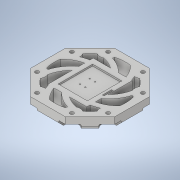
# Autodesk Inventor part: Bottom
Saved by Autodesk Inventor 2020 (Build 240168000, 168)
## iProperties
Created: 2018-10-03
Part Number: Bottom
Material: Generic
Document SubType Name: Modeling
Designer: isaac
Density: 1 g/cm^3
Appearance: Default
Author: isaac
Autodesk Inventor part; units mm, degrees
ref_plane "YZ Plane" through (0, 0, 0) normal (1, 0, 0) x (0, 1, 0)
ref_plane "XZ Plane" through (0, 0, 0) normal (0, 1, 0) x (-1, 0, 0)
ref_plane "XY Plane" through (0, 0, 0) normal (0, 0, 1) x (1, 0, 0)
sketch "Sketch1" plane through (0, 0, 0) normal (0, 1, 0) x (-1, 0, 0)
  circle A0 centre (0, 0) radius 88.9
  line L0 (82.1329, -34.0206) -> (34.0206, -82.1329)
  line L1 (34.0206, -82.1329) -> (-34.0206, -82.1329)
  line L2 (-34.0206, -82.1329) -> (-82.1329, -34.0206)
  line L3 (-82.1329, -34.0206) -> (-82.1329, 34.0206)
  line L4 (-82.1329, 34.0206) -> (-34.0206, 82.1329)
  line L5 (-34.0206, 82.1329) -> (34.0206, 82.1329)
  line L6 (34.0206, 82.1329) -> (82.1329, 34.0206)
  line L7 (82.1329, 34.0206) -> (82.1329, -34.0206)
  line L8 (0, 0) -> (105.0624, 0)
  line L9 (0, 0) -> (82.1329, 0)
  dimension "d0" = 177.8
  dimension "d1" = 68.0411
  constraints: 20 end point, 2 coincident, 1 collinear, 1 horizontal, 1 midpoint, 20 other
  measures "d1" distance of L0.end L1.end
extrude "Extrusion1" add sketch "Sketch1" along normal blind 25.4 contours L7 L0 L1 L2 L3 L4 L5 L6
sketch "Sketch31" plane through (0, 25.4, 0) normal (0, 1, 0) x (1, 0, 0)
  circle A0 centre (34.0206, 69.4329) radius 3.6195
  line L0 (34.0206, 82.1329) -> (-34.0206, 82.1329) projected
  line L1 (0, 0) -> (89.8026, 89.8026)
  line L2 (0, 0) -> (127, 0) construction
  circle A1 centre (69.4329, 34.0206) radius 3.6195
  circle A2 centre (-69.4329, 34.0206) radius 3.6195
  circle A3 centre (-34.0206, 69.4329) radius 3.6195
  circle A4 centre (-34.0206, -69.4329) radius 3.6195
  circle A5 centre (-69.4329, -34.0206) radius 3.6195
  circle A6 centre (69.4329, -34.0206) radius 3.6195
  circle A7 centre (34.0206, -69.4329) radius 3.6195
  dimension "d212" = 7.239
  dimension "d213" = 12.7
  dimension "d214" = 0
  dimension "d215" = 127
  dimension "d216" = 45
  dimension "d219" = 360
  constraints: 8 centre point, 4 end point, 1 equal length, 1 horizontal, 1 symmetric about line, 18 other
  measures "d212" diameter of A0
  measures "d213" distance from line of L0 A0.centre
  measures "d214" horizontal distance of L0.start A0.centre
  measures "d215" distance of L1.start L1.end
  measures "d216" angle of L2 L1
chamfer "Chamfer17" distance 8.89 angle 45 9 edges at (82.1329, 0, 0) (58.0767, 0, 58.0767) (0, 0, 82.1329) (-58.0767, 0, 58.0767) (-82.1329, 0, 17.0103) (-82.1329, 0, -17.0103) (-58.0767, 0, -58.0767) (0, 0, -82.1329) (58.0767, 0, -58.0767)
extrude "Extrusion26" cut sketch "Sketch31" against normal blind 25.4
sketch "Sketch32" plane through (0, 0, 0) normal (0, -1, 0) x (1, 0, 0)
  circle A0 centre (69.4329, 34.0206) radius 3.6195 projected
  circle A1 centre (69.4329, 34.0206) radius 12.7
  circle A2 centre (34.0206, 69.4329) radius 3.6195 projected
  circle A3 centre (34.0206, 69.4329) radius 12.7
  circle A4 centre (-34.0206, 69.4329) radius 12.7
  circle A5 centre (-69.4329, 34.0206) radius 12.7
  circle A6 centre (-69.4329, -34.0206) radius 12.7
  circle A7 centre (-34.0206, -69.4329) radius 12.7
  circle A8 centre (34.0206, -69.4329) radius 12.7
  circle A9 centre (69.4329, -34.0206) radius 12.7
  line L0 (69.4329, 21.3206) -> (90.8174, 21.3206)
  line L1 (36.643, 66.9381) -> (66.9381, 36.643) projected
  line L2 (60.5167, 43.0644) -> (77.7137, 60.0187)
  line L3 (77.7137, 60.0187) -> (96.7746, 43.8668)
  line L4 (96.7746, 43.8668) -> (90.8174, 21.3206)
  line L5 (43.0644, 60.5167) -> (60.2704, 77.969)
  line L6 (60.2704, 77.969) -> (26.119, 108.2881)
  line L7 (21.3206, 69.4329) -> (21.3206, 92.0788)
  line L8 (21.3206, 92.0788) -> (26.119, 108.2881)
  circle A10 centre (-34.0206, 69.4329) radius 12.7
  circle A11 centre (-69.4329, 34.0206) radius 12.7
  line L9 (-69.4329, 21.3206) -> (-92.0788, 21.3206)
  line L10 (-60.5167, 43.0644) -> (-77.969, 60.2704)
  line L11 (-92.0788, 21.3206) -> (-108.2881, 26.119)
  line L12 (-43.0644, 60.5167) -> (-60.0187, 77.7137)
  line L13 (-77.969, 60.2704) -> (-108.2881, 26.119)
  line L14 (-21.3206, 69.4329) -> (-21.3206, 90.8174)
  line L15 (-60.0187, 77.7137) -> (-43.8668, 96.7746)
  line L16 (-43.8668, 96.7746) -> (-21.3206, 90.8174)
  circle A12 centre (-69.4329, -34.0206) radius 12.7
  circle A13 centre (-34.0206, -69.4329) radius 12.7
  line L17 (-21.3206, -69.4329) -> (-21.3206, -92.0788)
  line L18 (-43.0644, -60.5167) -> (-60.2704, -77.969)
  line L19 (-21.3206, -92.0788) -> (-26.119, -108.2881)
  line L20 (-60.5167, -43.0644) -> (-77.7137, -60.0187)
  line L21 (-60.2704, -77.969) -> (-26.119, -108.2881)
  line L22 (-69.4329, -21.3206) -> (-90.8174, -21.3206)
  line L23 (-77.7137, -60.0187) -> (-96.7746, -43.8668)
  line L24 (-96.7746, -43.8668) -> (-90.8174, -21.3206)
  circle A14 centre (34.0206, -69.4329) radius 12.7
  circle A15 centre (69.4329, -34.0206) radius 12.7
  line L25 (69.4329, -21.3206) -> (92.0788, -21.3206)
  line L26 (60.5167, -43.0644) -> (77.969, -60.2704)
  line L27 (92.0788, -21.3206) -> (108.2881, -26.119)
  line L28 (43.0644, -60.5167) -> (60.0187, -77.7137)
  line L29 (77.969, -60.2704) -> (108.2881, -26.119)
  line L30 (21.3206, -69.4329) -> (21.3206, -90.8174)
  line L31 (60.0187, -77.7137) -> (43.8668, -96.7746)
  line L32 (43.8668, -96.7746) -> (21.3206, -90.8174)
  point P0 (0, 0)
  dimension "d226" = 25.4
  dimension "d227" = 25.4
  dimension "d230" = 360
  dimension "d291" = 360
  constraints: 64 end point, 16 point on circle, 14 centre point, 2 coincident, 2 point on line, 2 tangent, 1 horizontal, 1 vertical, 108 other
  measures "d226" diameter of A1
  measures "d227" diameter of A3
extrude "Extrusion27" cut sketch "Sketch32" against normal blind 12.7 contours A0 | A1 | A1 L2 L3 L4 L0 | A2 | A3 | A3 L7 L8 L6 L5 | A4 | A4 L12 L15 L16 L14 | A5 | A5 L9 L11 L13 L10 | A6 | A6 L20 L23 L24 L22 | A7 | L17 L19 L21 L18 A7 | A8 | A8 L28 L31 L32 L30 | A9 | A9 L25 L27 L29 L26
sketch "Sketch33" plane through (0, 25.4, 0) normal (0, 1, 0) x (1, 0, 0)
  line L0 (-28.575, 33.655) -> (28.575, 33.655)
  line L1 (28.575, 33.655) -> (28.575, -33.655)
  line L2 (28.575, -33.655) -> (-28.575, -33.655)
  line L3 (-28.575, -33.655) -> (-28.575, 33.655)
  line L4 (-28.575, 33.655) -> (28.575, -33.655) construction
  line L5 (28.575, 33.655) -> (-28.575, -33.655) construction
  point P0 (0, 0)
  dimension "d234" = 57.15
  dimension "d235" = 67.31
  constraints: 12 end point, 2 midpoint, 2 parallel, 1 horizontal, 1 perpendicular
  measures "d234" distance of L1.end L2.end
  measures "d235" distance of L0.end L1.end
extrude "Extrusion28" cut sketch "Sketch33" against normal blind 3.175
sketch "Sketch35" plane through (0, 25.4, 0) normal (0, 1, 0) x (1, 0, 0)
  line L0 (-82.1329, 34.0206) -> (-82.1329, -34.0206) projected
  line L1 (-34.0206, 82.1329) -> (-82.1329, 34.0206) projected
  line L2 (34.0206, 82.1329) -> (-34.0206, 82.1329) projected
  line L3 (49.3059, 66.8475) -> (66.8475, 49.3059) projected
  line L4 (82.1329, -34.0206) -> (82.1329, 34.0206) projected
  line L5 (66.8475, -49.3059) -> (49.3059, -66.8475) projected
  line L6 (21.3206, -82.1329) -> (-21.3206, -82.1329) projected
  line L7 (-49.3059, -66.8475) -> (-66.8475, -49.3059) projected
  arc A0 (-38.1, 9.1271) -> (-58.2083, -22.7945) centre (4.8156, -40.2008) ccw
  line L8 (-38.1, -44.45) -> (38.1, -44.45)
  line L9 (-38.1, -44.45) -> (38.1, 44.45) construction
  line L10 (38.1, -44.45) -> (-38.1, 44.45) construction
  arc A1 (2.7863, 44.45) -> (-22.7945, 58.2083) centre (-40.2008, -4.8156) ccw
  arc A2 (41.3, -6.1494) -> (58.2083, 22.7945) centre (-4.8156, 40.2008) ccw
  arc A3 (-2.7863, -44.45) -> (11.3195, -53.8433) centre (40.2008, 4.8156) ccw
  arc A4 (11.0921, 44.45) -> (-19.42, 63.2007) centre (-40.2008, -4.8156) ccw
  arc A5 (38.1, -16.5117) -> (63.2007, 19.42) centre (-4.8156, 40.2008) ccw
  arc A6 (-11.0921, -44.45) -> (19.42, -63.2007) centre (40.2008, 4.8156) ccw
  arc A7 (-38.1, 16.5117) -> (-63.2007, -19.42) centre (4.8156, -40.2008) ccw
  arc A8 (-38.1, 38.0757) -> (-53.574, 33.3053) centre (-25.0211, -31.8314) ccw
  arc A9 (36.5833, 44.45) -> (33.3053, 53.574) centre (-31.8314, 25.0211) ccw
  arc A10 (38.1, -38.0757) -> (53.574, -33.3053) centre (25.0211, 31.8314) ccw
  arc A11 (-36.5833, -44.45) -> (-33.3053, -53.574) centre (31.8314, -25.0211) ccw
  circle A12 centre (-69.4329, 34.0206) radius 3.6195 projected
  circle A13 centre (-34.0206, 69.4329) radius 3.6195 projected
  circle A14 centre (34.0206, 69.4329) radius 3.6195 projected
  circle A15 centre (69.4329, -34.0206) radius 3.6195 projected
  circle A16 centre (34.0206, -69.4329) radius 3.6195 projected
  circle A17 centre (-34.0206, -69.4329) radius 3.6195 projected
  circle A18 centre (-69.4329, -34.0206) radius 3.6195 projected
  arc A19 (25.9496, 44.45) -> (10.8089, 68.5864) centre (-31.8314, 25.0211) ccw
  arc A20 (38.1, -3.0933) -> (54.8559, 27.7335) centre (-4.8156, 40.2008) ccw
  arc A21 (38.1, -27.7091) -> (68.5864, -10.8089) centre (25.0211, 31.8314) ccw
  arc A22 (4.2978, -44.45) -> (27.7335, -54.8559) centre (40.2008, 4.8156) ccw
  arc A23 (-25.9496, -44.45) -> (-10.8089, -68.5864) centre (31.8314, -25.0211) ccw
  arc A24 (-38.1, 3.0933) -> (-54.8559, -27.7335) centre (4.8156, -40.2008) ccw
  arc A25 (-38.1, 27.7091) -> (-68.5864, 10.8089) centre (-25.0211, -31.8314) ccw
  arc A26 (-40.3622, 31.7268) -> (-55.8284, 25.8392) centre (-25.0211, -31.8314) ccw
  arc A27 (-66.9456, 18.3416) -> (-66.9727, 18.3189) centre (-25.0211, -31.8314) ccw
  arc A28 (-53.574, 33.3053) -> (-55.5293, 41.6825) centre (-69.4329, 34.0206) ccw
  arc A29 (-41.6825, 55.5293) -> (-55.5293, 41.6825) centre (0, 0) ccw
  arc A30 (-19.42, 63.2007) -> (-18.3382, 66.9674) centre (-34.0206, 69.4329) ccw
  arc A31 (-24.4956, 82.1329) -> (-49.6272, 66.5263) centre (-34.0206, 69.4329) ccw
  arc A32 (-41.6825, 55.5293) -> (-27.7335, 54.8559) centre (-34.0206, 69.4329) ccw
  arc A33 (-66.9674, 18.3382) -> (-66.9674, -18.3382) centre (0, 0) ccw
  arc A34 (-55.5293, -41.6825) -> (-66.9674, -18.3382) centre (-69.4329, -34.0206) ccw
  arc A35 (-82.1329, -24.4956) -> (-66.5263, -49.6272) centre (-69.4329, -34.0206) ccw
  arc A36 (-66.5263, 49.6272) -> (-82.1329, 24.4956) centre (-69.4329, 34.0206) ccw
  arc A37 (-66.9674, 18.3382) -> (-55.8284, 25.8392) centre (-69.4329, 34.0206) ccw
  arc A38 (-55.5293, -41.6825) -> (-41.6825, -55.5293) centre (0, 0) ccw
  arc A39 (-30.5986, -44.45) -> (-25.8392, -55.8284) centre (31.8314, -25.0211) ccw
  arc A40 (-18.3416, -66.9456) -> (-18.3189, -66.9727) centre (31.8314, -25.0211) ccw
  arc A41 (-49.6272, -66.5263) -> (-24.4956, -82.1329) centre (-34.0206, -69.4329) ccw
  arc A42 (-18.3382, -66.9674) -> (-18.3416, -66.9456) centre (-34.0206, -69.4329) ccw
  arc A43 (-33.3053, -53.574) -> (-41.6825, -55.5293) centre (-34.0206, -69.4329) ccw
  arc A44 (-18.3382, -66.9674) -> (-18.3189, -66.9727) centre (0, 0) ccw
  arc A45 (-10.8089, -68.5864) -> (18.3382, -66.9674) centre (0, 0) ccw
  arc A46 (24.4956, -82.1329) -> (49.6272, -66.5263) centre (34.0206, -69.4329) ccw
  arc A47 (41.6825, -55.5293) -> (27.7335, -54.8559) centre (34.0206, -69.4329) ccw
  arc A48 (19.42, -63.2007) -> (18.3382, -66.9674) centre (34.0206, -69.4329) ccw
  arc A49 (41.6825, -55.5293) -> (55.5293, -41.6825) centre (0, 0) ccw
  arc A50 (66.5263, -49.6272) -> (82.1329, -24.4956) centre (69.4329, -34.0206) ccw
  arc A51 (38.1, -32.2306) -> (55.8284, -25.8392) centre (25.0211, 31.8314) ccw
  arc A52 (66.9456, -18.3416) -> (66.9727, -18.3189) centre (25.0211, 31.8314) ccw
  line L11 (38.1, -44.45) -> (38.1, -38.0757)
  arc A53 (66.9674, -18.3382) -> (55.8284, -25.8392) centre (69.4329, -34.0206) ccw
  arc A54 (53.574, -33.3053) -> (55.5293, -41.6825) centre (69.4329, -34.0206) ccw
  arc A55 (66.9674, -18.3382) -> (66.9727, -18.3189) centre (0, 0) ccw
  arc A56 (68.5864, -10.8089) -> (66.9674, 18.3382) centre (0, 0) ccw
  arc A57 (63.2007, 19.42) -> (66.9674, 18.3382) centre (69.4329, 34.0206) ccw
  arc A58 (82.1329, 24.4956) -> (66.5263, 49.6272) centre (69.4329, 34.0206) ccw
  arc A59 (55.5293, 41.6825) -> (54.8559, 27.7335) centre (69.4329, 34.0206) ccw
  line L12 (38.1, -32.2306) -> (38.1, -16.5117)
  line L13 (38.1, -3.0933) -> (38.1, 44.45)
  arc A60 (55.5293, 41.6825) -> (41.6825, 55.5293) centre (0, 0) ccw
  arc A61 (18.3382, 66.9674) -> (-18.3382, 66.9674) centre (0, 0) ccw
  arc A62 (30.5986, 44.45) -> (25.8392, 55.8284) centre (-31.8314, 25.0211) ccw
  arc A63 (18.3416, 66.9456) -> (18.3189, 66.9727) centre (-31.8314, 25.0211) ccw
  arc A64 (49.6272, 66.5263) -> (24.4956, 82.1329) centre (34.0206, 69.4329) ccw
  arc A65 (18.3382, 66.9674) -> (41.6825, 55.5293) centre (34.0206, 69.4329) ccw
  arc A66 (-4.2978, 44.45) -> (-27.7335, 54.8559) centre (-40.2008, -4.8156) ccw
  line L14 (38.1, 44.45) -> (2.7863, 44.45)
  line L15 (-4.2978, 44.45) -> (-38.1, 44.45)
  line L16 (-38.1, 3.0933) -> (-38.1, -44.45)
  line L17 (-38.1, 44.45) -> (-38.1, 38.0757)
  line L18 (-38.1, 27.7091) -> (-38.1, 16.5117)
  point P0 (46.7206, 69.4329)
  point P1 (69.4329, 46.7206)
  point P2 (69.4329, -46.7206)
  point P3 (46.7206, -69.4329)
  point P4 (34.0206, -82.1329)
  point P5 (-34.0206, -82.1329)
  point P6 (-46.7206, -69.4329)
  point P7 (-69.4329, -46.7206)
  dimension "d250" = 76.2
  dimension "d251" = 88.9
  dimension "d254" = 71.12
  dimension "d255" = 71.12
  dimension "d257" = 71.12
  dimension "d259" = 71.12
  dimension "d268" = 60.96
  dimension "d269" = 60.96
  dimension "d270" = 60.96
  dimension "d271" = 60.96
  dimension "d272" = 60.96
  dimension "d273" = 60.96
  dimension "d274" = 60.96
  dimension "d275" = 60.96
  constraints: 135 point on circle, 60 centre point, 27 point on line, 24 coincident, 22 end point, 11 parallel, 3 perpendicular, 1 horizontal, 1 midpoint
  measures "d250" distance of L10.end L9.end
  measures "d251" distance of L9.end L8.end
  measures "d254" radius of A4
  measures "d255" radius of A5
  measures "d257" radius of A6
  measures "d259" radius of A7
  measures "d268" radius of A19
  measures "d269" radius of A20
  measures "d270" radius of A21
  measures "d271" radius of A22
  measures "d272" radius of A23
  measures "d273" radius of A24
  measures "d274" radius of A25
  measures "d275" radius of A66
extrude "Extrusion30" cut sketch "Sketch35" against normal through all contours L8 A11 A43 A38 A34 A24 L16 | L8 A6 A48 A45 A23 | L8 L11 A10 A54 A49 A47 A22 | A4 A30 A61 A19 L14 | A9 A65 A60 A59 A20 L13 L14 | A5 A57 A56 A21 L12 | A7 A34 A33 A25 L18 | A8 A28 A29 A32 A66 L15 L17
fillet "Fillet5" radius 1.5875 8 edges at (-57.6824, 12.7, 29.2022) (-29.2022, 12.7, 57.6824) (29.2022, 12.7, 57.6824) (57.6824, 12.7, 29.2022) (-57.6824, 12.7, -29.2022) (-29.2022, 12.7, -57.6824) (29.2022, 12.7, -57.6824) (57.6824, 12.7, -29.2022)
fillet "Fillet6" radius 6.35 8 edges at (53.4874, 0, 0.5277) (35.1, 0, -49.0679) (-2.9644, 0, -55.7774) (-45.9732, 0, -36.1323) (-53.4874, 0, -0.5277) (-35.1, 0, 49.0679) (2.9644, 0, 55.7774) (45.9732, 0, 36.1323)
sketch "Sketch37" plane through (0, 0, 0) normal (0, -1, 0) x (1, 0, 0)
  circle A0 centre (-10.0076, 9.4933) radius 1.0351 construction
  circle A1 centre (-10.0076, -9.4933) radius 1.0351 construction
  circle A2 centre (0.4572, -9.4933) radius 1.0351 construction
  circle A3 centre (0.4572, 9.4933) radius 1.0351 construction
  circle A4 centre (0.4572, 9.4933) radius 1.143
  circle A5 centre (0.4572, -9.4933) radius 1.143
  circle A6 centre (-10.0076, -9.4933) radius 1.143
  circle A7 centre (-10.0076, 9.4933) radius 1.143
  point P0 (0, 0)
  dimension "d293" = 2.286
  constraints: 4 centre point, 4 coincident, 3 equal radius
  measures "d293" diameter of A4
extrude "Extrusion31" cut sketch "Sketch37" against normal through all
sketch "Sketch38" plane through (0, 0, 0) normal (0, -1, 0) x (1, 0, 0)
  line L0 (-12.7, 13.97) -> (19.05, 13.97)
  line L1 (19.05, 13.97) -> (19.05, -13.97)
  line L2 (19.05, -13.97) -> (-12.7, -13.97)
  line L3 (-12.7, -13.97) -> (-12.7, 13.97)
  line L4 (-12.7, 13.97) -> (19.05, -13.97) construction
  line L5 (19.05, 13.97) -> (-12.7, -13.97) construction
  line L6 (0, 0) -> (3.175, 0) construction
  point P0 (1.5875, 0)
  dimension "d297" = 27.94
  dimension "d298" = 31.75
  dimension "d299" = 19.05
  constraints: 14 end point, 3 midpoint, 2 parallel, 2 perpendicular, 1 horizontal
  measures "d297" distance of L0.end L1.end
  measures "d298" distance of L1.end L2.end
  measures "d299" distance from line of L1 L6.start
extrude "Extrusion32" cut sketch "Sketch38" against normal blind 6.35
sketch "Sketch39" plane through (0, 0, 0) normal (0, 0, 1) x (1, 0, 0)
  line L0 (-0.6858, 6.35) -> (1.6002, 6.35) projected
  line L1 (-0.6858, 6.35) -> (1.6002, 6.35) projected
  line L2 (-11.1506, 6.35) -> (-8.8646, 6.35) projected
  line L3 (-11.1506, 6.35) -> (-8.8646, 6.35) projected
  line L4 (19.05, 6.35) -> (-12.7, 6.35) projected
  line L5 (-12.7, 6.35) -> (19.05, 6.35) projected
  line L6 (19.05, 6.35) -> (29.1593, 10.0295)
  line L7 (33.3375, 15.9965) -> (33.3375, 25.4)
  line L8 (28.575, 25.4) -> (28.575, 22.225) projected
  line L9 (28.575, 25.4) -> (28.575, 22.225) projected
  line L10 (38.1, 0) -> (54.8559, 0) projected
  line L11 (38.1, 25.4) -> (38.1, 0) projected
  line L12 (54.8559, 25.4) -> (38.1, 25.4) projected
  line L13 (54.8559, 25.4) -> (54.8559, 0) projected
  line L14 (38.1, 25.4) -> (28.575, 25.4) construction
  arc A0 (29.1593, 10.0295) -> (33.3375, 15.9965) centre (26.9875, 15.9965) ccw
  point P0 (0, 0)
  dimension "d302" = 110
  dimension "d303" = 6.35
  constraints: 6 end point, 2 perpendicular, 2 point on circle, 2 tangent, 1 centre point, 1 midpoint
  measures "d302" angle of L7 L6
  measures "d303" radius of A0
sketch "Sketch40" plane through (19.05, 0, -13.97) normal (-1, 0, 0) x (0, 0, 1)
  line L0 (27.94, 6.35) -> (0, 6.35) projected
  line L1 (5.08, 3.175) -> (22.86, 3.175)
  line L2 (22.86, 3.175) -> (22.86, 6.35)
  line L3 (22.86, 6.35) -> (5.08, 6.35)
  line L4 (5.08, 6.35) -> (5.08, 3.175)
  line L5 (5.08, 3.175) -> (22.86, 6.35) construction
  line L6 (22.86, 3.175) -> (5.08, 6.35) construction
  line L7 (13.97, 0) -> (13.97, 4.7625) construction
  point P0 (5.08, 6.35)
  dimension "d304" = 3.175
  dimension "d305" = 17.78
  constraints: 14 end point, 2 midpoint, 2 parallel, 2 perpendicular, 1 horizontal, 1 point on line
  measures "d304" distance of L3.end L1.start
  measures "d305" distance of L1.start L1.end
sweep "Sweep1" cut profiles "Sketch40" path "Sketch39" path curves L7 A0 L6 L4
fillet "Fillet7" radius 3.175 4 edges at (3.175, 0, 13.97) (-12.7, 0, 0) (3.175, 0, -13.97) (19.05, 0, 0)
body "Solid1"
